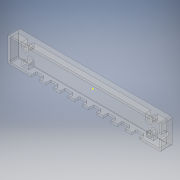
# Autodesk Inventor part: SH8_002.1-sunhub8-casing_top
Saved by Autodesk Inventor 2019 (Build 230136000, 136)
## iProperties
Created: 2019-02-22
Part Number: SH8_002.1-sunhub8-casing_top
Material: Generic
Document SubType Name: Modeling
Designer: Rene
Density: 1 g/cm^3
Appearance: Polycarbonate - Clear
Author: Rene
Autodesk Inventor part; units mm, degrees
ref_plane "YZ Plane" through (0, 0, 0) normal (1, 0, 0) x (0, 1, 0)
ref_plane "XZ Plane" through (0, 0, 0) normal (0, 1, 0) x (-1, 0, 0)
ref_plane "XY Plane" through (0, 0, 0) normal (0, 0, 1) x (1, 0, 0)
sketch "Sketch1" plane through (0, 0, 0) normal (0, 0, 1) x (1, 0, 0)
  line L0 (-107.5, -17.7) -> (107.5, -17.7)
  line L1 (107.5, -17.7) -> (107.5, 17.7)
  line L2 (107.5, 17.7) -> (-107.5, 17.7)
  line L3 (-107.5, 17.7) -> (-107.5, -17.7)
  point P0 (0, 0)
  dimension "d0" = 35.4
  dimension "d1" = 17.7
  dimension "d2" = 215
  dimension "d3" = 107.5
  constraints: 8 end point, 2 parallel, 1 horizontal, 1 perpendicular
  measures "d0" distance of L2.end L0.start
  measures "d1" vertical distance of point (0, 0) L0.start
  measures "d2" distance of L1.end L2.end
  measures "d3" horizontal distance of point (0, 0) L2.end
extrude "Extrusion1" add sketch "Sketch1" along normal blind 15
fillet "Fillet1" radius 2 4 edges at (-107.5, -17.7, 7.5) (-107.5, 17.7, 7.5) (107.5, -17.7, 7.5) (107.5, 17.7, 7.5)
sketch "Sketch2" plane through (0, 0, 15) normal (0, 0, 1) x (1, 0, 0)
  line L0 (-104.2, -14.7) -> (104.2, -14.7)
  line L1 (104.2, -14.7) -> (104.2, 14.7)
  line L2 (104.2, 14.7) -> (-104.2, 14.7)
  line L3 (-104.2, 14.7) -> (-104.2, -14.7)
  line L4 (105.5, 17.7) -> (-105.5, 17.7) projected
  line L5 (-105.5, -17.7) -> (105.5, -17.7) projected
  line L6 (-107.5, 15.7) -> (-107.5, -15.7) projected
  line L7 (107.5, -15.7) -> (107.5, 15.7) projected
  point P0 (0, 0)
  dimension "d7" = 3
  dimension "d8" = 3
  dimension "d9" = 3.3
  dimension "d10" = 3.3
  constraints: 8 end point, 2 parallel, 1 horizontal, 1 perpendicular
  measures "d7" distance between parallel lines of L4 L2
  measures "d8" distance between parallel lines of L5 L0
  measures "d9" distance between parallel lines of L3 L6
  measures "d10" distance between parallel lines of L7 L1
extrude "Extrusion2" cut sketch "Sketch2" against normal blind 11
sketch "Sketch4" plane through (107.5, -15.7, 0) normal (1, 0, 0) x (0, 0, -1)
  line L0 (-15, 1) -> (-15, 30.4) projected
  line L1 (-15, 18.95) -> (-5, 18.95)
  line L2 (-5, 18.95) -> (-5, 12.45)
  line L3 (-5, 12.45) -> (-15, 12.45)
  line L4 (-15, 12.45) -> (-15, 18.95)
  line L5 (0, 0) -> (0, 31.4) projected
  point P0 (0, 15.7)
  point P1 (-20, 19.45)
  dimension "d19" = 6.5
  dimension "d20" = 10
  dimension "d21" = 3.25
  constraints: 8 end point, 2 parallel, 1 horizontal, 1 perpendicular, 2 other
  measures "d19" distance between parallel lines of L1 L3
  measures "d20" distance of L2.end L3.end
  measures "d21" vertical distance of L1.end point (0, 15.7)
extrude "Extrusion4" cut sketch "Sketch4" against normal blind 20
fillet "Fillet2" radius 3.25 2 edges at (105.85, 3.25, 5) (105.85, -3.25, 5)
sketch "Sketch5" plane through (-105.5, -17.7, 0) normal (0, -1, 0) x (1, 0, 0)
  line L0 (0, 15) -> (211, 15) projected
  line L1 (182.2, 15) -> (171.2, 15)
  line L2 (171.2, 15) -> (171.2, 8)
  line L3 (171.2, 8) -> (182.2, 8)
  line L4 (182.2, 8) -> (182.2, 15)
  line L5 (213, 0) -> (213, 15) projected
  line L6 (209.7, 15) -> (209.7, 4) projected
  point P0 (105.5, 0)
  dimension "d23" = 7
  dimension "d24" = 11
  dimension "d32" = 27.5
  constraints: 8 end point, 2 parallel, 1 horizontal, 1 perpendicular, 1 point on line
  measures "d23" distance of L3.end L1.start
  measures "d24" distance of L2.end L3.end
  measures "d32" distance from line of L1.start L6
extrude "Extrusion5" cut sketch "Sketch5" against normal blind 5
fillet "Fillet3" radius 1 2 edges at (76.7, -16.2, 8) (65.7, -16.2, 8)
pattern_linear "Rectangular Pattern1" count 8 spacing 20 along (-1, 0, 0) of "Extrusion5", "Fillet3"
sketch "Sketch6" plane through (0, 0, 4) normal (0, 0, 1) x (1, 0, 0)
  line L0 (86.5, -9) -> (-86.5, -9) construction
  line L1 (-86.5, -9) -> (-86.5, 9) construction
  line L2 (-86.5, 9) -> (86.5, 9) construction
  line L3 (86.5, 9) -> (86.5, -9) construction
  circle A0 centre (86.5, -9) radius 2.3
  circle A1 centre (86.5, -9) radius 4.75
  circle A2 centre (86.5, 9) radius 2.3
  circle A3 centre (86.5, 9) radius 4.75
  circle A4 centre (-86.5, -9) radius 2.3
  circle A5 centre (-86.5, 9) radius 2.3
  circle A6 centre (-86.5, -9) radius 4.75
  circle A7 centre (-86.5, 9) radius 4.75
  point P0 (0, 0)
  dimension "d33" = 173
  dimension "d34" = 86.5
  dimension "d35" = 18
  dimension "d36" = 9
  dimension "d62" = 4.6
  dimension "d63" = 9.5
  dimension "d64" = 4.6
  dimension "d65" = 9.5
  dimension "d66" = 4.6
  dimension "d67" = 4.6
  dimension "d68" = 9.5
  dimension "d69" = 9.5
  constraints: 12 coincident, 8 centre point, 8 end point, 2 parallel, 1 horizontal, 1 perpendicular
  measures "d33" distance of L0.start L0.end
  measures "d34" horizontal distance of point (0, 0) L0.start
  measures "d35" distance of L2.end L0.start
  measures "d36" vertical distance of point (0, 0) L2.end
  measures "d62" diameter of A0
  measures "d63" diameter of A1
  measures "d64" diameter of A2
  measures "d65" diameter of A3
  measures "d66" diameter of A4
  measures "d67" diameter of A5
  measures "d68" diameter of A7
  measures "d69" diameter of A6
extrude "Extrusion6" add sketch "Sketch6" along normal blind 7.8
sketch "Sketch7" plane through (0, 0, 4) normal (0, 0, 1) x (1, 0, 0)
  circle A0 centre (86.5, -9) radius 4.75 projected
  line L0 (104.2, -14.7) -> (76.7, -14.7) projected
  line L1 (91.25, -9) -> (91.25, -14.7)
  line L2 (81.75, -9) -> (81.75, -14.7)
  point P0 (0, 0)
  constraints: 4 end point, 2 perpendicular, 2 point on circle, 2 point on line
extrude "Extrusion7" add sketch "Sketch7" along normal blind 6 contours L1 L0 L2 A0
mirror "Mirror1" about plane through (0, 0, 0) normal (0, 1, 0) of "Extrusion7"
mirror "Mirror2" about plane through (0, 0, 0) normal (1, 0, 0) of "Extrusion7", "Mirror1"
sketch "Sketch9" plane through (86.5, -9, 11.8) normal (0, 0, 1) x (1, 0, 0)
  circle A0 centre (0, 0) radius 4.75 projected
  circle A1 centre (0, 0) radius 3.75
  point P0 (-86.5, 9)
  dimension "d81" = 1
  constraints: 1 centre point
  measures "d81" radial gap between concentric circles of A0 A1
extrude "Extrusion9" cut sketch "Sketch9" against normal blind 1.8
sketch "Sketch10" plane through (-86.5, -9, 10) normal (0, 0, 1) x (1, 0, 0)
  arc A0 (-4.75, 0) -> (4.75, 0) centre (0, 0) ccw projected
  line L0 (-4.75, -5.7) -> (-4.75, 0) projected
  line L1 (4.75, -5.7) -> (-4.75, -5.7) projected
  line L2 (4.75, 0) -> (4.75, -5.7) projected
  point P0 (86.5, 9)
extrude "Extrusion10" add sketch "Sketch10" along normal blind 1.8
sketch "Sketch11" plane through (0, 0, 4) normal (0, 0, 1) x (1, 0, 0)
  point P0 (0, 0)
sketch "Sketch12" plane through (-86.5, 9, 10) normal (0, 0, 1) x (1, 0, 0)
  arc A0 (4.75, 0) -> (-4.75, 0) centre (0, 0) ccw projected
  line L0 (4.75, 0) -> (4.75, 5.7) projected
  line L1 (-4.75, 5.7) -> (4.75, 5.7) projected
  line L2 (-4.75, 5.7) -> (-4.75, 0) projected
  point P0 (86.5, -9)
extrude "Extrusion11" add sketch "Sketch12" along normal blind 1.8
sketch "Sketch13" plane through (86.5, 9, 10) normal (0, 0, 1) x (1, 0, 0)
  arc A0 (4.75, 0) -> (-4.75, 0) centre (0, 0) ccw projected
  line L0 (4.75, 5.7) -> (4.75, 0) projected
  line L1 (-4.75, 5.7) -> (4.75, 5.7) projected
  line L2 (-4.75, 0) -> (-4.75, 5.7) projected
  point P0 (-86.5, -9)
extrude "Extrusion12" add sketch "Sketch13" along normal blind 1.8
equation "\"d1\" = 0.5 * d0"
equation "\"d3\" = 0.5 * d2"
equation "\"d8\" = d7"
equation "\"d10\" = d9"
equation "\"d21\" = 0.5 * d19"
equation "\"d34\" = 0.5 * d33"
equation "\"d36\" = 0.5 * d35"
equation "\"d64\" = d62"
equation "\"d65\" = d63"
equation "\"d66\" = d62"
equation "\"d67\" = d62"
equation "\"d68\" = d63"
equation "\"d69\" = d63"
body "Solid1"
